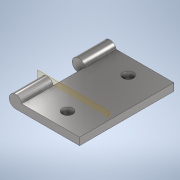
# Autodesk Inventor part: final right
Saved by Autodesk Inventor 2020 (Build 240168000, 168)
## iProperties
Created: 2021-03-06
Part Number: final right
Material: Stainless Steel
Document SubType Name: Modeling
Designer: Danish
Density: 8 g/cm^3
Appearance: Semi-Polished
Author: Danish
Autodesk Inventor part; units mm, degrees
ref_plane "YZ Plane" through (0, 0, 0) normal (1, 0, 0) x (0, 1, 0)
ref_plane "XZ Plane" through (0, 0, 0) normal (0, 1, 0) x (-1, 0, 0)
ref_plane "XY Plane" through (0, 0, 0) normal (0, 0, 1) x (1, 0, 0)
sketch "Sketch11" plane through (0, 0, 0) normal (0, 0, 1) x (1, 0, 0)
  line L0 (0, 0) -> (27.764, 0)
  line L1 (27.764, 0) -> (27.764, 3.519)
  line L2 (27.764, 3.519) -> (0, 3.519)
  line L3 (0, 3.519) -> (0, 0)
  circle A0 centre (0, 3) radius 3
  point P0 (2.9548, 3.519)
  dimension "d25" = 27.764
  dimension "d26" = 3.519
  dimension "d27" = 6
  constraints: 8 end point, 2 parallel, 1 centre point, 1 horizontal, 1 perpendicular
  measures "d25" distance of L2.end L1.end
  measures "d26" distance of L1.end L0.end
  measures "d27" diameter of A0
extrude "Extrusion5" add sketch "Sketch11" along normal blind 45
ref_plane "Work Plane3" through (0, 0, 30) normal (0, 0, 1) x (1, 0, 0)
sketch "Sketch12" plane through (0, 0, 30) normal (0, 0, 1) x (1, 0, 0)
  circle A0 centre (0, 3) radius 3
  point P0 (0, 0)
  dimension "d32" = 6
  constraints: 1 centre point
  measures "d32" diameter of A0
extrude "Extrusion6" cut sketch "Sketch12" against normal blind 15
sketch "Sketch13" plane through (27.764, 0, 0) normal (1, 0, 0) x (0, 0, -1)
  point P0 (0, 0)
sketch "Sketch14" plane through (2.9548, 3.519, 0) normal (0, 1, 0) x (1, 0, 0)
  line L0 (24.8092, 0) -> (24.8092, -45) projected
  line L1 (24.8092, 0) -> (30.3097, 0)
  line L2 (30.3097, 0) -> (30.3097, -45)
  line L3 (30.3097, -45) -> (24.8092, -45)
  line L4 (24.8092, -45) -> (24.8092, 0)
  point P0 (-2.9548, 0)
  dimension "d35" = 45
  constraints: 8 end point, 2 parallel, 1 horizontal, 1 perpendicular
  measures "d35" distance of L1.end L2.end
extrude "Extrusion7" add sketch "Sketch14" against normal blind 3.5
sketch "Sketch15" plane through (2.9548, 3.519, 15) normal (0, 1, 0) x (1, 0, 0)
  line L0 (30.3097, 15) -> (30.3097, -30) projected
  line L1 (24.8092, 15) -> (30.3097, 15) projected
  line L2 (30.3097, -30) -> (27.5595, -30)
  line L3 (27.5595, -30) -> (27.5595, 15)
  line L4 (27.5595, 15) -> (30.3097, 15)
  line L5 (30.3097, 15) -> (30.3097, -30)
  point P0 (-2.9548, 15)
  constraints: 8 end point, 2 parallel, 1 horizontal, 1 midpoint, 1 perpendicular
extrude "Extrusion8" cut sketch "Sketch15" against normal blind 3.5
sketch "Sketch16" plane through (1.0163, 3.519, 45.1466) normal (0, 1, 0) x (1, 0, 0)
  point P0 (-2.9547, 45)
  point P1 (15.912, 7.9951)
  point P2 (15.5243, 37.2981)
hole "Hole2" at (16.9284, 3.519, 37.1515) at (16.5406, 3.519, 7.8485) direction (0, -1, 0) diameter 5 end through all
body "Solid2"
